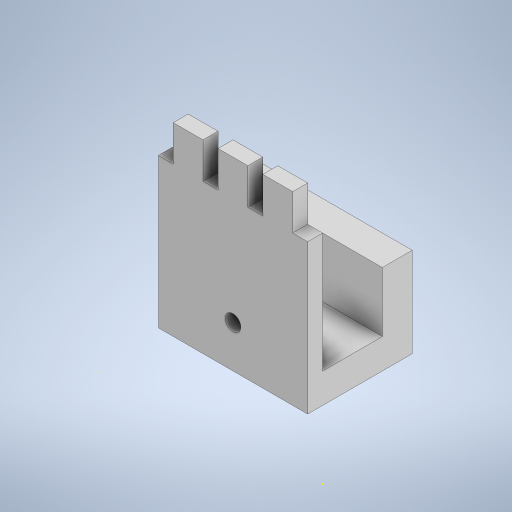
# Autodesk Inventor part: Casis Kiri Roda
Saved by Autodesk Inventor 2023 (Build 270158000, 158)
## iProperties
Created: 2025-05-21
Part Number: Casis Kiri Roda
Material: Generic
Document SubType Name: Modeling
Designer: ASUS
Density: 1 g/cm^3
Appearance: Default
Author: ASUS
Autodesk Inventor part; units mm, degrees
ref_plane "YZ Plane" through (0, 0, 0) normal (1, 0, 0) x (0, 1, 0)
ref_plane "XZ Plane" through (0, 0, 0) normal (0, 1, 0) x (-1, 0, 0)
ref_plane "XY Plane" through (0, 0, 0) normal (0, 0, 1) x (1, 0, 0)
sketch "Sketch1" plane through (0, 0, 0) normal (0, 0, 1) x (1, 0, 0)
  line L0 (69.608, 72.6391) -> (69.608, 22.6391)
  line L1 (69.608, 22.6391) -> (19.608, 22.6391)
  line L2 (19.608, 22.6391) -> (19.608, 72.6391)
  line L3 (19.608, 72.6391) -> (24.608, 72.6391)
  line L4 (24.608, 72.6391) -> (24.608, 84.6391)
  line L5 (24.608, 84.6391) -> (34.608, 84.6391)
  line L6 (34.608, 84.6391) -> (34.608, 72.6391)
  line L7 (34.608, 72.6391) -> (39.608, 72.6391)
  line L8 (39.608, 72.6391) -> (39.608, 84.6391)
  line L9 (39.608, 84.6391) -> (49.608, 84.6391)
  line L10 (49.608, 84.6391) -> (49.608, 72.6391)
  line L11 (49.608, 72.6391) -> (54.608, 72.6391)
  line L12 (54.608, 72.6391) -> (54.608, 84.6391)
  line L13 (54.608, 84.6391) -> (64.608, 84.6391)
  line L14 (64.608, 84.6391) -> (64.608, 72.6391)
  line L15 (64.608, 72.6391) -> (69.608, 72.6391)
  point P0 (0, 0)
  dimension "d0" = 50
  dimension "d1" = 50
  dimension "d2" = 5
  dimension "d3" = 12
  dimension "d4" = 10
  dimension "d5" = 12
  dimension "d6" = 5
  dimension "d7" = 12
  dimension "d8" = 10
  dimension "d9" = 12
  dimension "d10" = 5
  dimension "d11" = 12
  dimension "d12" = 10
  dimension "d13" = 12
  dimension "d14" = 5
  constraints: 32 end point, 7 perpendicular, 3 point on line, 2 vertical, 1 horizontal, 1 parallel
  measures "d0" distance of L0.end L1.end
  measures "d1" distance of L0.start L0.end
  measures "d2" distance of L2.end L3.end
  measures "d3" distance of L3.end L4.end
  measures "d4" distance of L4.end L5.end
  measures "d5" distance of L5.end L6.end
  measures "d6" distance of L6.end L7.end
  measures "d7" distance of L7.end L8.end
  measures "d8" distance of L8.end L9.end
  measures "d9" distance of L9.end L10.end
  measures "d10" distance of L10.end L11.end
  measures "d11" distance of L11.end L12.end
  measures "d12" distance of L12.end L13.end
  measures "d13" distance of L13.end L14.end
  measures "d14" distance of L14.end L0.start
extrude "Extrusion1" add sketch "Sketch1" along normal blind 5
sketch "Sketch2" plane through (69.608, 22.6391, 0) normal (1, 0, 0) x (0, 0, -1)
  line L0 (0, 50) -> (0, 0) projected
  line L1 (0, 0) -> (30, 0)
  line L2 (30, 0) -> (30, 25)
  line L3 (30, 25) -> (20, 25)
  line L4 (20, 25) -> (20, 10)
  line L5 (20, 10) -> (0, 10)
  point P0 (0, -22.6391)
  dimension "d17" = 30
  dimension "d18" = 25
  dimension "d19" = 10
  dimension "d20" = 15
  dimension "d21" = 20
  constraints: 10 end point, 2 horizontal, 2 perpendicular, 1 point on line
  measures "d17" distance of L0.end L1.end
  measures "d18" distance of L1.end L2.end
  measures "d19" distance of L2.end L3.end
  measures "d20" distance of L3.end L4.end
  measures "d21" distance of L4.end L5.end
sketch "Sketch3" plane through (0, 0, 5) normal (0, 0, 1) x (1, 0, 0)
  point P0 (0, 0)
extrude "Extrusion2" add sketch "Sketch2" against normal blind 50
sketch "Sketch4" plane through (69.608, 22.6391, 5) normal (1, 0, 0) x (0, 0, -1)
  line L0 (35, 25) -> (25, 25) projected
  line L1 (35, 25) -> (35, 30)
  line L2 (35, 25) -> (35, 0) projected
  line L3 (35, 30) -> (25, 30)
  line L4 (25, 30) -> (25, 25)
  line L5 (25, 25) -> (35, 25)
  point P0 (5, -22.6391)
  dimension "d24" = 5
  dimension "d25" = 10
  dimension "d26" = 5
  dimension "d27" = 10
  constraints: 8 end point, 2 perpendicular, 1 collinear
  measures "d24" distance of L0.start L1.end
  measures "d25" distance of L1.end L3.end
  measures "d26" distance of L3.end L4.end
  measures "d27" distance of L4.end L0.start
extrude "Extrusion3" add sketch "Sketch4" against normal blind 50
sketch "Sketch5" plane through (69.608, 22.6391, 5) normal (1, 0, 0) x (0, 0, -1)
  point P0 (5, -22.6391)
sketch "Sketch6" plane through (0, 0, 5) normal (0, 0, 1) x (1, 0, 0)
  line L0 (69.608, 22.6391) -> (19.608, 22.6391) projected
  circle A0 centre (44.608, 36.6391) radius 2.65
  point P0 (0, 0)
  dimension "d31" = 5.3
  constraints: 1 centre point
  measures "d31" diameter of A0
extrude "Extrusion4" cut sketch "Sketch6" against normal blind 50
sketch "Sketch7" plane through (69.608, 22.6391, 5) normal (1, 0, 0) x (0, 0, -1)
  point P0 (5, -22.6391)
sketch "Sketch8" plane through (0, 0, 5) normal (0, 0, 1) x (1, 0, 0)
  point P0 (0, 0)
sketch "Sketch9" plane through (69.608, 22.6391, 5) normal (1, 0, 0) x (0, 0, -1)
  point P0 (5, -22.6391)
sketch "Sketch10" plane through (69.608, 22.6391, 5) normal (1, 0, 0) x (0, 0, -1)
  point P0 (5, -22.6391)
body "Solid1"
